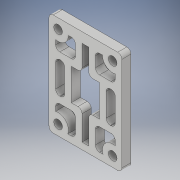
# Autodesk Inventor part: LED Riser
Saved by Autodesk Inventor 2017.3 (Build 213256000, 256)
## iProperties
Created: 2019-07-16
Part Number: LED Riser
Material: Generic
Document SubType Name: Modeling
Designer: LSabe
Density: 1 g/cm^3
Appearance: Default
Author: LSabe
Autodesk Inventor part; units mm, degrees
ref_plane "YZ Plane" through (0, 0, 0) normal (1, 0, 0) x (0, 1, 0)
ref_plane "XZ Plane" through (0, 0, 0) normal (0, 1, 0) x (-1, 0, 0)
ref_plane "XY Plane" through (0, 0, 0) normal (0, 0, 1) x (1, 0, 0)
sketch "Sketch1" plane through (0, 0, 0) normal (0, 0, 1) x (1, 0, 0)
  line L0 (-3.81, -7.6835) -> (45.466, -7.6835)
  line L1 (48.641, -4.5085) -> (48.641, 67.2465)
  line L2 (45.466, 70.4215) -> (-3.81, 70.4215)
  line L3 (-6.985, 67.2465) -> (-6.985, -4.5085)
  arc A0 (45.466, -7.6835) -> (48.641, -4.5085) centre (45.466, -4.5085) ccw
  arc A1 (-6.985, -4.5085) -> (-3.81, -7.6835) centre (-3.81, -4.5085) ccw
  line L4 (31.623, 19.304) -> (31.623, 43.434)
  line L5 (10.033, 43.434) -> (10.033, 19.304)
  line L6 (18.288, -7.6835) -> (23.368, -7.6835)
  line L7 (23.368, 70.4215) -> (18.288, 70.4215)
  arc A2 (-1.905, 55.0979) -> (7.874, 62.738) centre (0, 62.738) ccw
  arc A3 (33.782, 62.738) -> (43.561, 55.0979) centre (41.656, 62.738) ccw
  arc A4 (43.561, 7.6401) -> (34.2249, -2.6035) centre (41.656, 0) ccw
  arc A5 (7.4311, -2.6035) -> (-1.905, 7.6401) centre (0, 0) ccw
  line L8 (34.2249, -2.6035) -> (31.623, -2.6035)
  line L9 (10.033, -2.6035) -> (7.4311, -2.6035)
  line L10 (31.623, 43.434) -> (26.543, 43.434)
  line L11 (15.113, 43.434) -> (10.033, 43.434)
  line L12 (10.033, 19.304) -> (15.113, 19.304)
  line L13 (26.543, 19.304) -> (31.623, 19.304)
  line L14 (23.368, 46.609) -> (23.368, 62.738)
  line L15 (18.288, 62.738) -> (18.288, 46.609)
  line L16 (23.368, -2.6035) -> (23.368, 16.129)
  line L17 (18.288, 16.129) -> (18.288, -2.6035)
  line L18 (18.288, -2.6035) -> (23.368, -2.6035)
  line L19 (28.448, 51.689) -> (28.448, 59.563)
  line L20 (40.386, 48.514) -> (31.623, 48.514)
  line L21 (13.208, 59.563) -> (13.208, 51.689)
  line L22 (10.033, 48.514) -> (1.27, 48.514)
  line L23 (13.208, 11.049) -> (13.208, 0.5715)
  line L24 (1.27, 14.224) -> (10.033, 14.224)
  line L25 (31.623, 14.224) -> (40.386, 14.224)
  line L26 (28.448, 0.5715) -> (28.448, 11.049)
  line L27 (-1.905, 7.6401) -> (-1.905, 11.049)
  line L28 (-1.905, 51.689) -> (-1.905, 55.0979)
  line L29 (43.561, 55.0979) -> (43.561, 51.689)
  line L30 (43.561, 11.049) -> (43.561, 7.6401)
  line L31 (43.561, 22.479) -> (43.561, 40.259)
  line L32 (-1.905, 40.259) -> (-1.905, 22.479)
  line L33 (4.953, 40.259) -> (4.953, 22.479)
  line L34 (36.703, 22.479) -> (36.703, 40.259)
  line L35 (1.27, 43.434) -> (1.778, 43.434)
  line L36 (1.778, 19.304) -> (1.27, 19.304)
  line L37 (39.878, 43.434) -> (40.386, 43.434)
  line L38 (40.386, 19.304) -> (39.878, 19.304)
  arc A6 (10.033, 48.514) -> (13.208, 51.689) centre (10.033, 51.689) ccw
  arc A7 (28.448, 51.689) -> (31.623, 48.514) centre (31.623, 51.689) ccw
  arc A8 (31.623, 14.224) -> (28.448, 11.049) centre (31.623, 11.049) ccw
  arc A9 (13.208, 11.049) -> (10.033, 14.224) centre (10.033, 11.049) ccw
  arc A10 (1.27, 14.224) -> (-1.905, 11.049) centre (1.27, 11.049) ccw
  arc A11 (10.033, -2.6035) -> (13.208, 0.5715) centre (10.033, 0.5715) ccw
  arc A12 (28.448, 0.5715) -> (31.623, -2.6035) centre (31.623, 0.5715) ccw
  arc A13 (43.561, 11.049) -> (40.386, 14.224) centre (40.386, 11.049) ccw
  arc A14 (40.386, 48.514) -> (43.561, 51.689) centre (40.386, 51.689) ccw
  arc A15 (-1.905, 51.689) -> (1.27, 48.514) centre (1.27, 51.689) ccw
  arc A16 (23.368, 46.609) -> (26.543, 43.434) centre (26.543, 46.609) ccw
  arc A17 (15.113, 43.434) -> (18.288, 46.609) centre (15.113, 46.609) ccw
  arc A18 (18.288, 16.129) -> (15.113, 19.304) centre (15.113, 16.129) ccw
  arc A19 (26.543, 19.304) -> (23.368, 16.129) centre (26.543, 16.129) ccw
  arc A20 (36.703, 22.479) -> (39.878, 19.304) centre (39.878, 22.479) ccw
  arc A21 (40.386, 19.304) -> (43.561, 22.479) centre (40.386, 22.479) ccw
  arc A22 (43.561, 40.259) -> (40.386, 43.434) centre (40.386, 40.259) ccw
  arc A23 (39.878, 43.434) -> (36.703, 40.259) centre (39.878, 40.259) ccw
  arc A24 (1.27, 43.434) -> (-1.905, 40.259) centre (1.27, 40.259) ccw
  arc A25 (4.953, 40.259) -> (1.778, 43.434) centre (1.778, 40.259) ccw
  arc A26 (1.778, 19.304) -> (4.953, 22.479) centre (1.778, 22.479) ccw
  arc A27 (-1.905, 22.479) -> (1.27, 19.304) centre (1.27, 22.479) ccw
  line L39 (7.874, 62.738) -> (10.033, 62.738)
  line L40 (18.288, 62.738) -> (23.368, 62.738)
  line L41 (31.623, 62.738) -> (33.782, 62.738)
  arc A28 (13.208, 59.563) -> (10.033, 62.738) centre (10.033, 59.563) ccw
  arc A29 (31.623, 62.738) -> (28.448, 59.563) centre (31.623, 59.563) ccw
  circle A30 centre (0, 62.738) radius 3.302
  circle A31 centre (41.656, 62.738) radius 3.302
  circle A32 centre (0, 0) radius 3.302
  circle A33 centre (41.656, 0) radius 3.302
  arc A34 (-3.81, 70.4215) -> (-6.985, 67.2465) centre (-3.81, 67.2465) ccw
  arc A35 (48.641, 67.2465) -> (45.466, 70.4215) centre (45.466, 67.2465) ccw
  point P0 (20.828, 31.369)
  point P1 (-6.985, 70.4215)
  point P2 (48.641, 70.4215)
  point P3 (23.368, 43.434)
  point P4 (18.288, 43.434)
  point P5 (18.288, 19.304)
  point P6 (23.368, 19.304)
  point P7 (-1.905, 14.224)
  point P8 (43.561, 48.514)
  point P9 (43.561, 14.224)
  point P10 (-1.905, 48.514)
  point P11 (13.208, 65.3415)
  point P12 (28.448, 65.3415)
  point P13 (13.208, -2.6035)
  point P14 (28.448, -2.6035)
  point P15 (28.448, 48.514)
  point P16 (13.208, 48.514)
  point P17 (13.208, 14.224)
  point P18 (28.448, 14.224)
  point P19 (-1.905, 19.304)
  point P20 (43.561, 43.434)
  point P21 (43.561, 19.304)
  point P22 (-1.905, 43.434)
  point P23 (4.953, 43.434)
  point P24 (4.953, 19.304)
  point P25 (36.703, 19.304)
  point P26 (36.703, 43.434)
  point P27 (28.448, 62.738)
  point P28 (13.208, 62.738)
  dimension "d32" = 3.175
  dimension "d37" = 6.604
  dimension "d38" = 6.604
  dimension "d39" = 6.604
  dimension "d40" = 6.604
  dimension "d76" = 3.175
  constraints: 84 end point, 64 point on circle, 56 point on line, 56 tangent, 36 centre point, 31 parallel, 22 equal radius, 12 horizontal, 9 perpendicular, 4 coincident
  measures "d32" radius of A28
  measures "d37" diameter of A30
  measures "d38" diameter of A31
  measures "d39" diameter of A32
  measures "d40" diameter of A33
  measures "d76" radius of A34
extrude "Extrusion1" add sketch "Sketch1" along normal blind 6.985
body "Solid1"
